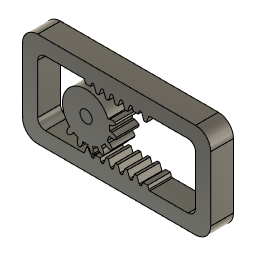
movement-114 v32 (Autodesk Fusion 360 design; units mm, degrees)
description: Spur Gear; Module: 2.0; Num Teeth: 18; Pressure Angle: 20.0; Backlash: 0.15 mm
Autodesk Fusion 360 part; units mm, degrees
note: some values were not read from the file. Set by a fixed rule: which face or edge a step refers to.
sketch "rack-side" plane through (0, 0, 0) normal (0, 1, 0) x (1, 0, 0)
  line L0 (0, 0) -> (43.9823, 0)
  line L1 (43.9823, 0) -> (43.9823, -10)
  line L2 (43.9823, -10) -> (0, -10)
  line L3 (0, -10) -> (0, 0)
  line L4 (0, -12.5) -> (43.9823, -12.5) construction
  line L5 (0, -14.5) -> (43.9823, -14.5) construction
  line L6 (0.6609, -10) -> (2.2987, -14.5)
  line L7 (2.2987, -14.5) -> (3.9844, -14.5)
  line L8 (3.9844, -14.5) -> (5.6223, -10)
  line L9 (0, -31.25) -> (43.9823, -31.25) construction
  point P0 (1.5708, -12.5)
  point P1 (4.7124, -12.5)
  point P2 (3.1416, -14.5)
  point P3 (21.9911, -31.25)
  dimension "d8" = 43.9823
  dimension "d9" = 10
  dimension "d10" = 2.5
  dimension "d11" = 2
  dimension "d12" = 70
  dimension "d13" = 3.1416
  dimension "d14" = 3.1416
  dimension "d32" = 18.75
  constraint horizontal L0
  constraint vertical L1
  constraint horizontal L2
  constraint vertical L3
  constraint coincident L0.start L3.end
  constraint coincident L3 L5.start
  constraint coincident L3 L4.start
  constraint equal L2 L4
  constraint equal L2 L5
  constraint coincident L2 L6.start
  constraint coincident L5 L6.end
  constraint coincident L5 L7.end
  constraint coincident L2 L8.end
  constraint equal L6 L8
  constraint coincident L4 P0
  constraint coincident L6 P0
  constraint coincident L8 P1
  constraint coincident L4 P1
  constraint midpoint L7 P2
  constraint horizontal L9
  constraint coincident L3 L9.start
  constraint equal L0 L9
  constraint midpoint L9 P3
  measures "d8" distance of L0.start L0.end
  measures "d9" distance of L0.start L2.end
  measures "d10" distance of L2 L4
  measures "d11" distance of L4 L5
  measures "d12" angle of L2 L6
  measures "d13" distance of P0 P1
  measures "d14" distance of L3 P2
  measures "d32" distance of L4 L9
extrude "Extrude1" add sketch "rack-side" along normal blind 15 contours L0 L1 L2 L3 makes body 1
extrude "Extrude2" add sketch "rack-side" along normal blind 15 contours L2 L6 L7 L8 bodies 1
fillet "Fillet1" radius 0.76 2 edges at (0.6609, 7.5, 10) (5.6223, 7.5, 10) on bodies 1
pattern_linear "R-Pattern1" count 7 spacing 6.2832 along (1, 0, 0) of "Extrude2", "Fillet1"
copy_body "Body->Comp1" bodies 1 removing the originals makes body 2 in component "rack"
ref_plane "WorkPlane1" through (21.9911, 7.5, 5) normal (-1, 0, 0) x (0, 0, 1) in component "rack"
ref_plane "WorkPlane2" through (21.9911, 0, 31.25) normal (0, 0, 1) x (1, 0, 0) in component "rack"
extrude "Extrude1'" add 1 faces at (0, 5, 6.6667) along direction (-1, 0, 0) blind 40 on bodies 2 bodies 2 in component "rack"
mirror "Mirror1" about plane through (21.9911, 7.5, 5) normal (-1, 0, 0) of "Extrude1'" in component "rack"
mirror "Mirror2" about plane through (21.9911, 0, 31.25) normal (0, 0, 1) of bodies 2 makes body 3 in component "rack"
sketch "rack-top" plane through (0, 0, 10) normal (0, 0, 1) x (-1, 0, 0)
  line L0 (-0.1287, 0) -> (-0.1287, -15)
  line L1 (-0.1287, -15) -> (40, -15)
  line L2 (40, -15) -> (40, 0)
  line L3 (40, 0) -> (-0.1287, 0)
  line L4 (-0.1287, -15) -> (40, -15)
  line L5 (40, 0) -> (40, -15)
  line L6 (-0.1287, -15) -> (-0.1287, 0)
  line L7 (-0.1287, 0) -> (40, 0)
  line L8 (30, -15) -> (30, 0)
  dimension "d35" = 10
  constraint coincident L4 L8.start
  constraint coincident L7 L8.end
  constraint perpendicular L7 L8
  measures "d35" distance of L5 L8
extrude "Extrude2'" add sketch "rack-top" along normal up to surface (42.5 mm away) contours L1 L2 L3 L4 L5 L7 L8 bodies 2 3 in component "rack"
mirror "Mirror3" about plane through (21.9911, 7.5, 5) normal (-1, 0, 0) of "Extrude2'" in component "rack"
fillet "Fillet1'" radius 10 4 edges at (83.9823, 7.5, 62.5) (83.9823, 7.5, 0) (-40, 7.5, 0) (-40, 7.5, 62.5) on bodies 2 in component "rack"
fillet "Fillet2" radius 5 4 edges at (73.9823, 7.5, 10) (73.9823, 7.5, 52.5) (-30, 7.5, 52.5) (-30, 7.5, 10) on bodies 2 in component "rack"
ref_plane "WorkPlane3" through (21.9911, 7.5, 31.25) normal (0, 0, 1) x (-1, 0, 0)
sketch "Sketch1" plane through (0, 0, 0) normal (0, 0, 1) x (1, 0, 0) in component "spur-gear"
  circle A0 centre (0, 0) radius 15.5492
extrude "Extrude1''" add sketch "Sketch1" along normal blind 15 separate body makes body 4 in component "spur-gear"
sketch "Sketch2" plane through (0, 0, 0) normal (0, 0, 1) x (1, 0, 0) in component "spur-gear"
  spline S0 degree 5 poles (16.8298, -1.6901) (16.8389, -1.691) (16.8569, -1.6926) (16.8841, -1.6941) (16.9204, -1.6949) (16.9658, -1.6938) (17.0113, -1.6914) (17.0569, -1.6881) (17.1025, -1.6843) (17.1481, -1.6802) (17.1937, -1.6757) (17.2394, -1.6708) (17.2851, -1.6653) (17.3308, -1.6592) (17.3764, -1.6524) (17.4221, -1.6449) (17.4678, -1.6369) (17.5136, -1.6284) (17.5593, -1.6195) (17.605, -1.6103) (17.6507, -1.6007) (17.6963, -1.5906) (17.742, -1.5802) (17.7877, -1.5693) (17.8334, -1.5581) (17.879, -1.5464) (17.9246, -1.5343) (17.9703, -1.5218) (18.0159, -1.509) (18.0614, -1.4958) (18.107, -1.4823) (18.1525, -1.4685) (18.1981, -1.4543) (18.2436, -1.4397) (18.289, -1.4249) (18.3345, -1.4096) (18.3799, -1.3941) (18.4253, -1.3782) (18.4707, -1.362) (18.516, -1.3455) (18.5613, -1.3287) (18.6066, -1.3116) (18.6518, -1.2941) (18.697, -1.2764) (18.7422, -1.2584) (18.7874, -1.24) (18.8325, -1.2214) (18.8775, -1.2024) (18.9226, -1.1832) (18.9676, -1.1637) (19.0125, -1.1439) (19.0574, -1.1238) (19.1023, -1.1035) (19.1471, -1.0828) (19.1919, -1.0619) (19.2367, -1.0407) (19.2814, -1.0192) (19.326, -0.9975) (19.3706, -0.9755) (19.4152, -0.9532) (19.4597, -0.9307) (19.5041, -0.9079) (19.5485, -0.8848) (19.5929, -0.8615) (19.6372, -0.8379) (19.6815, -0.814) (19.7257, -0.7899) (19.7698, -0.7655) (19.8139, -0.7409) (19.858, -0.7161) (19.902, -0.6909) (19.9371, -0.6706) (19.9634, -0.6553) (19.981, -0.645) (19.9898, -0.6399) knots 0 0 0 0 0 0 0.01428571 0.02857143 0.04285714 0.05714286 0.07142857 0.08571429 0.1 0.11428571 0.12857143 0.14285714 0.15714286 0.17142857 0.18571429 0.2 0.21428571 0.22857143 0.24285714 0.25714286 0.27142857 0.28571429 0.3 0.31428571 0.32857143 0.34285714 0.35714286 0.37142857 0.38571429 0.4 0.41428571 0.42857143 0.44285714 0.45714286 0.47142857 0.48571429 0.5 0.51428571 0.52857143 0.54285714 0.55714286 0.57142857 0.58571429 0.6 0.61428571 0.62857143 0.64285714 0.65714286 0.67142857 0.68571429 0.7 0.71428571 0.72857143 0.74285714 0.75714286 0.77142857 0.78571429 0.8 0.81428571 0.82857143 0.84285714 0.85714286 0.87142857 0.88571429 0.9 0.91428571 0.92857143 0.94285714 0.95714286 0.97142857 0.98571429 1 1 1 1 1 1
  spline S1 degree 5 poles (16.8298, 1.6901) (16.8389, 1.691) (16.8569, 1.6926) (16.8841, 1.6941) (16.9204, 1.6949) (16.9658, 1.6938) (17.0113, 1.6914) (17.0569, 1.6881) (17.1025, 1.6843) (17.1481, 1.6802) (17.1937, 1.6757) (17.2394, 1.6708) (17.2851, 1.6653) (17.3308, 1.6592) (17.3764, 1.6524) (17.4221, 1.6449) (17.4678, 1.6369) (17.5136, 1.6284) (17.5593, 1.6195) (17.605, 1.6103) (17.6507, 1.6007) (17.6963, 1.5906) (17.742, 1.5802) (17.7877, 1.5693) (17.8334, 1.5581) (17.879, 1.5464) (17.9246, 1.5343) (17.9703, 1.5218) (18.0159, 1.509) (18.0614, 1.4958) (18.107, 1.4823) (18.1525, 1.4685) (18.1981, 1.4543) (18.2436, 1.4397) (18.289, 1.4249) (18.3345, 1.4096) (18.3799, 1.3941) (18.4253, 1.3782) (18.4707, 1.362) (18.516, 1.3455) (18.5613, 1.3287) (18.6066, 1.3116) (18.6518, 1.2941) (18.697, 1.2764) (18.7422, 1.2584) (18.7874, 1.24) (18.8325, 1.2214) (18.8775, 1.2024) (18.9226, 1.1832) (18.9676, 1.1637) (19.0125, 1.1439) (19.0574, 1.1238) (19.1023, 1.1035) (19.1471, 1.0828) (19.1919, 1.0619) (19.2367, 1.0407) (19.2814, 1.0192) (19.326, 0.9975) (19.3706, 0.9755) (19.4152, 0.9532) (19.4597, 0.9307) (19.5041, 0.9079) (19.5485, 0.8848) (19.5929, 0.8615) (19.6372, 0.8379) (19.6815, 0.814) (19.7257, 0.7899) (19.7698, 0.7655) (19.8139, 0.7409) (19.858, 0.7161) (19.902, 0.6909) (19.9371, 0.6706) (19.9634, 0.6553) (19.981, 0.645) (19.9898, 0.6399) knots 0 0 0 0 0 0 0.01428571 0.02857143 0.04285714 0.05714286 0.07142857 0.08571429 0.1 0.11428571 0.12857143 0.14285714 0.15714286 0.17142857 0.18571429 0.2 0.21428571 0.22857143 0.24285714 0.25714286 0.27142857 0.28571429 0.3 0.31428571 0.32857143 0.34285714 0.35714286 0.37142857 0.38571429 0.4 0.41428571 0.42857143 0.44285714 0.45714286 0.47142857 0.48571429 0.5 0.51428571 0.52857143 0.54285714 0.55714286 0.57142857 0.58571429 0.6 0.61428571 0.62857143 0.64285714 0.65714286 0.67142857 0.68571429 0.7 0.71428571 0.72857143 0.74285714 0.75714286 0.77142857 0.78571429 0.8 0.81428571 0.82857143 0.84285714 0.85714286 0.87142857 0.88571429 0.9 0.91428571 0.92857143 0.94285714 0.95714286 0.97142857 0.98571429 1 1 1 1 1 1
  arc A0 (19.9898, -0.6399) -> (19.9898, 0.6399) centre (0, 0) ccw
  line L0 (15.4614, -1.5537) -> (16.8298, -1.6901)
  line L1 (15.4614, 1.5537) -> (16.8298, 1.6901)
  line L2 (15.4614, -1.5537) -> (15.4614, 1.5537)
  point P0 (17.0515, -1.6884)
  point P1 (17.2751, -1.6664)
  point P2 (17.4998, -1.6309)
  point P3 (17.7254, -1.5839)
  point P4 (17.9516, -1.5269)
  point P5 (18.1783, -1.4604)
  point P6 (18.4052, -1.3852)
  point P7 (18.6322, -1.3017)
  point P8 (18.8592, -1.2101)
  point P9 (19.0861, -1.1108)
  point P10 (19.3127, -1.0039)
  point P11 (19.539, -0.8897)
  point P12 (19.7647, -0.7683)
  point P13 (17.0515, 1.6884)
  point P14 (17.2751, 1.6664)
  point P15 (17.4998, 1.6309)
  point P16 (17.7254, 1.5839)
  point P17 (17.9516, 1.5269)
  point P18 (18.1783, 1.4604)
  point P19 (18.4052, 1.3852)
  point P20 (18.6322, 1.3017)
  point P21 (18.8592, 1.2101)
  point P22 (19.0861, 1.1108)
  point P23 (19.3127, 1.0039)
  point P24 (19.539, 0.8897)
  point P25 (19.7647, 0.7683)
extrude "Extrude2''" add sketch "Sketch2" along normal blind 15 bodies 4 in component "spur-gear"
pattern_circular "C-Pattern1" count 15 over 360 about axis through (0, 0, 0) along (0, 0, 1) of "Extrude2''" in component "spur-gear"
sketch "Sketch3" plane through (0, 0, 0) normal (0, 0, 1) x (1, 0, 0) in component "spur-gear"
  circle A0 centre (0, 0) radius 18 construction
  circle A1 centre (0, 0) radius 4
  dimension "d73_1" = 8
  constraint concentric A0 A1
  constraint coincident A0.centre A1.centre
  measures "d73_1" diameter of A1
extrude "Extrude3" cut sketch "Sketch3" along normal through all bodies 4 in component "spur-gear"
sketch "Sketch1 (2)" plane through (0, 0, 0) normal (0, 1, 0) x (1, 0, 0) in component "shaft"
  circle A0 centre (4.7674, -31.1301) radius 4
extrude "Extrude1'''" add sketch "Sketch1 (2)" along normal blind 50 separate body makes body 5 in component "shaft"
move_body "Move1" bodies 5 to x (1, 0, 0) y (0, 1, 0) z (0, 0, 1) at (-20, -5, 0) in component "shaft"
move_face "OffsetFaces7" offset -2 4 faces at (40.5598, 5, 14.5) (9.1438, 5, 14.5) (2.8606, 5, 48) (34.2766, 5, 48) on bodies 2 in component "rack"
sketch "Sketch7" plane through (0, 0, 0) normal (0, 0, 1) x (1, 0, 0) in component "spur-gear"
  circle A0 centre (0, 0) radius 15.5492
  line L0 (-14.81, -4.7374) -> (-16.1107, -5.1523)
  spline S0 degree 5 poles (-16.1107, -5.1523) (-16.1193, -5.155) (-16.1367, -5.1603) (-16.1629, -5.1675) (-16.1983, -5.1758) (-16.2429, -5.1842) (-16.2879, -5.1913) (-16.3332, -5.1975) (-16.3786, -5.2033) (-16.4241, -5.2087) (-16.4696, -5.2139) (-16.5153, -5.2186) (-16.5611, -5.2227) (-16.6071, -5.2262) (-16.6532, -5.229) (-16.6994, -5.2312) (-16.7458, -5.2329) (-16.7923, -5.2341) (-16.8388, -5.2349) (-16.8855, -5.2354) (-16.9322, -5.2355) (-16.9789, -5.2352) (-17.0258, -5.2344) (-17.0727, -5.2333) (-17.1197, -5.2318) (-17.1668, -5.2298) (-17.2139, -5.2275) (-17.2612, -5.2248) (-17.3084, -5.2217) (-17.3557, -5.2183) (-17.4031, -5.2146) (-17.4506, -5.2105) (-17.498, -5.2061) (-17.5456, -5.2013) (-17.5931, -5.1962) (-17.6408, -5.1908) (-17.6884, -5.185) (-17.7361, -5.1789) (-17.7839, -5.1725) (-17.8316, -5.1658) (-17.8795, -5.1588) (-17.9273, -5.1514) (-17.9752, -5.1438) (-18.0231, -5.1358) (-18.071, -5.1276) (-18.119, -5.119) (-18.167, -5.1102) (-18.215, -5.101) (-18.2631, -5.0916) (-18.3111, -5.0819) (-18.3592, -5.0718) (-18.4073, -5.0615) (-18.4554, -5.0509) (-18.5036, -5.0401) (-18.5517, -5.0289) (-18.5999, -5.0175) (-18.6481, -5.0058) (-18.6963, -4.9938) (-18.7445, -4.9816) (-18.7927, -4.969) (-18.8409, -4.9562) (-18.8892, -4.9432) (-18.9374, -4.9298) (-18.9857, -4.9162) (-19.0339, -4.9024) (-19.0821, -4.8882) (-19.1304, -4.8738) (-19.1787, -4.8592) (-19.2269, -4.8443) (-19.2752, -4.8291) (-19.3234, -4.8137) (-19.362, -4.8011) (-19.3909, -4.7916) (-19.4102, -4.7852) (-19.4199, -4.782) knots 0 0 0 0 0 0 0.01428571 0.02857143 0.04285714 0.05714286 0.07142857 0.08571429 0.1 0.11428571 0.12857143 0.14285714 0.15714286 0.17142857 0.18571429 0.2 0.21428571 0.22857143 0.24285714 0.25714286 0.27142857 0.28571429 0.3 0.31428571 0.32857143 0.34285714 0.35714286 0.37142857 0.38571429 0.4 0.41428571 0.42857143 0.44285714 0.45714286 0.47142857 0.48571429 0.5 0.51428571 0.52857143 0.54285714 0.55714286 0.57142857 0.58571429 0.6 0.61428571 0.62857143 0.64285714 0.65714286 0.67142857 0.68571429 0.7 0.71428571 0.72857143 0.74285714 0.75714286 0.77142857 0.78571429 0.8 0.81428571 0.82857143 0.84285714 0.85714286 0.87142857 0.88571429 0.9 0.91428571 0.92857143 0.94285714 0.95714286 0.97142857 0.98571429 1 1 1 1 1 1
  arc A1 (-19.686, -3.5302) -> (-19.4199, -4.782) centre (0, 0) ccw
  spline S1 degree 5 poles (-16.8134, -1.8459) (-16.8225, -1.8469) (-16.8405, -1.8492) (-16.8674, -1.8533) (-16.903, -1.8601) (-16.9473, -1.8706) (-16.9913, -1.8824) (-17.0351, -1.8952) (-17.0789, -1.9083) (-17.1227, -1.9219) (-17.1664, -1.9357) (-17.2101, -1.95) (-17.2536, -1.9648) (-17.297, -1.9803) (-17.3403, -1.9965) (-17.3834, -2.0133) (-17.4265, -2.0307) (-17.4694, -2.0485) (-17.5123, -2.0666) (-17.555, -2.0852) (-17.5977, -2.1041) (-17.6403, -2.1234) (-17.6829, -2.1431) (-17.7253, -2.1632) (-17.7676, -2.1838) (-17.8098, -2.2047) (-17.8519, -2.226) (-17.894, -2.2477) (-17.9359, -2.2697) (-17.9778, -2.292) (-18.0195, -2.3147) (-18.0612, -2.3377) (-18.1028, -2.3611) (-18.1442, -2.3848) (-18.1856, -2.4088) (-18.2269, -2.4331) (-18.2681, -2.4578) (-18.3092, -2.4827) (-18.3502, -2.508) (-18.3911, -2.5336) (-18.432, -2.5595) (-18.4727, -2.5856) (-18.5133, -2.6121) (-18.5539, -2.6388) (-18.5943, -2.6659) (-18.6346, -2.6932) (-18.6749, -2.7208) (-18.715, -2.7487) (-18.7551, -2.7769) (-18.795, -2.8053) (-18.8349, -2.834) (-18.8746, -2.863) (-18.9143, -2.8922) (-18.9539, -2.9217) (-18.9933, -2.9515) (-19.0327, -2.9816) (-19.0719, -3.0118) (-19.1111, -3.0424) (-19.1501, -3.0732) (-19.1891, -3.1042) (-19.2279, -3.1356) (-19.2667, -3.1671) (-19.3053, -3.1989) (-19.3439, -3.231) (-19.3823, -3.2633) (-19.4206, -3.2958) (-19.4589, -3.3286) (-19.497, -3.3616) (-19.535, -3.3948) (-19.5729, -3.4283) (-19.6107, -3.462) (-19.6409, -3.4892) (-19.6634, -3.5096) (-19.6785, -3.5233) (-19.686, -3.5302) knots 0 0 0 0 0 0 0.01428571 0.02857143 0.04285714 0.05714286 0.07142857 0.08571429 0.1 0.11428571 0.12857143 0.14285714 0.15714286 0.17142857 0.18571429 0.2 0.21428571 0.22857143 0.24285714 0.25714286 0.27142857 0.28571429 0.3 0.31428571 0.32857143 0.34285714 0.35714286 0.37142857 0.38571429 0.4 0.41428571 0.42857143 0.44285714 0.45714286 0.47142857 0.48571429 0.5 0.51428571 0.52857143 0.54285714 0.55714286 0.57142857 0.58571429 0.6 0.61428571 0.62857143 0.64285714 0.65714286 0.67142857 0.68571429 0.7 0.71428571 0.72857143 0.74285714 0.75714286 0.77142857 0.78571429 0.8 0.81428571 0.82857143 0.84285714 0.85714286 0.87142857 0.88571429 0.9 0.91428571 0.92857143 0.94285714 0.95714286 0.97142857 0.98571429 1 1 1 1 1 1
  line L1 (-15.4564, -1.696) -> (-16.8134, -1.8459)
  line L2 (-15.4564, 1.696) -> (-16.8134, 1.8459)
  spline S2 degree 5 poles (-16.8134, 1.8459) (-16.8225, 1.8469) (-16.8405, 1.8492) (-16.8674, 1.8533) (-16.903, 1.8601) (-16.9473, 1.8706) (-16.9913, 1.8824) (-17.0351, 1.8952) (-17.0789, 1.9083) (-17.1227, 1.9219) (-17.1664, 1.9357) (-17.2101, 1.95) (-17.2536, 1.9648) (-17.297, 1.9803) (-17.3403, 1.9965) (-17.3834, 2.0133) (-17.4265, 2.0307) (-17.4694, 2.0485) (-17.5123, 2.0666) (-17.555, 2.0852) (-17.5977, 2.1041) (-17.6403, 2.1234) (-17.6829, 2.1431) (-17.7253, 2.1632) (-17.7676, 2.1838) (-17.8098, 2.2047) (-17.8519, 2.226) (-17.894, 2.2477) (-17.9359, 2.2697) (-17.9778, 2.292) (-18.0195, 2.3147) (-18.0612, 2.3377) (-18.1028, 2.3611) (-18.1442, 2.3848) (-18.1856, 2.4088) (-18.2269, 2.4331) (-18.2681, 2.4578) (-18.3092, 2.4827) (-18.3502, 2.508) (-18.3911, 2.5336) (-18.432, 2.5595) (-18.4727, 2.5856) (-18.5133, 2.6121) (-18.5539, 2.6388) (-18.5943, 2.6659) (-18.6346, 2.6932) (-18.6749, 2.7208) (-18.715, 2.7487) (-18.7551, 2.7769) (-18.795, 2.8053) (-18.8349, 2.834) (-18.8746, 2.863) (-18.9143, 2.8922) (-18.9539, 2.9217) (-18.9933, 2.9515) (-19.0327, 2.9816) (-19.0719, 3.0118) (-19.1111, 3.0424) (-19.1501, 3.0732) (-19.1891, 3.1042) (-19.2279, 3.1356) (-19.2667, 3.1671) (-19.3053, 3.1989) (-19.3439, 3.231) (-19.3823, 3.2633) (-19.4206, 3.2958) (-19.4589, 3.3286) (-19.497, 3.3616) (-19.535, 3.3948) (-19.5729, 3.4283) (-19.6107, 3.462) (-19.6409, 3.4892) (-19.6634, 3.5096) (-19.6785, 3.5233) (-19.686, 3.5302) knots 0 0 0 0 0 0 0.01428571 0.02857143 0.04285714 0.05714286 0.07142857 0.08571429 0.1 0.11428571 0.12857143 0.14285714 0.15714286 0.17142857 0.18571429 0.2 0.21428571 0.22857143 0.24285714 0.25714286 0.27142857 0.28571429 0.3 0.31428571 0.32857143 0.34285714 0.35714286 0.37142857 0.38571429 0.4 0.41428571 0.42857143 0.44285714 0.45714286 0.47142857 0.48571429 0.5 0.51428571 0.52857143 0.54285714 0.55714286 0.57142857 0.58571429 0.6 0.61428571 0.62857143 0.64285714 0.65714286 0.67142857 0.68571429 0.7 0.71428571 0.72857143 0.74285714 0.75714286 0.77142857 0.78571429 0.8 0.81428571 0.82857143 0.84285714 0.85714286 0.87142857 0.88571429 0.9 0.91428571 0.92857143 0.94285714 0.95714286 0.97142857 0.98571429 1 1 1 1 1 1
  arc A2 (-19.4199, 4.782) -> (-19.686, 3.5302) centre (0, 0) ccw
  spline S3 degree 5 poles (-16.1107, 5.1523) (-16.1193, 5.155) (-16.1367, 5.1603) (-16.1629, 5.1675) (-16.1983, 5.1758) (-16.2429, 5.1842) (-16.2879, 5.1913) (-16.3332, 5.1975) (-16.3786, 5.2033) (-16.4241, 5.2087) (-16.4696, 5.2139) (-16.5153, 5.2186) (-16.5611, 5.2227) (-16.6071, 5.2262) (-16.6532, 5.229) (-16.6994, 5.2312) (-16.7458, 5.2329) (-16.7923, 5.2341) (-16.8388, 5.2349) (-16.8855, 5.2354) (-16.9322, 5.2355) (-16.9789, 5.2352) (-17.0258, 5.2344) (-17.0727, 5.2333) (-17.1197, 5.2318) (-17.1668, 5.2298) (-17.2139, 5.2275) (-17.2612, 5.2248) (-17.3084, 5.2217) (-17.3557, 5.2183) (-17.4031, 5.2146) (-17.4506, 5.2105) (-17.498, 5.2061) (-17.5456, 5.2013) (-17.5931, 5.1962) (-17.6408, 5.1908) (-17.6884, 5.185) (-17.7361, 5.1789) (-17.7839, 5.1725) (-17.8316, 5.1658) (-17.8795, 5.1588) (-17.9273, 5.1514) (-17.9752, 5.1438) (-18.0231, 5.1358) (-18.071, 5.1276) (-18.119, 5.119) (-18.167, 5.1102) (-18.215, 5.101) (-18.2631, 5.0916) (-18.3111, 5.0819) (-18.3592, 5.0718) (-18.4073, 5.0615) (-18.4554, 5.0509) (-18.5036, 5.0401) (-18.5517, 5.0289) (-18.5999, 5.0175) (-18.6481, 5.0058) (-18.6963, 4.9938) (-18.7445, 4.9816) (-18.7927, 4.969) (-18.8409, 4.9562) (-18.8892, 4.9432) (-18.9374, 4.9298) (-18.9857, 4.9162) (-19.0339, 4.9024) (-19.0821, 4.8882) (-19.1304, 4.8738) (-19.1787, 4.8592) (-19.2269, 4.8443) (-19.2752, 4.8291) (-19.3234, 4.8137) (-19.362, 4.8011) (-19.3909, 4.7916) (-19.4102, 4.7852) (-19.4199, 4.782) knots 0 0 0 0 0 0 0.01428571 0.02857143 0.04285714 0.05714286 0.07142857 0.08571429 0.1 0.11428571 0.12857143 0.14285714 0.15714286 0.17142857 0.18571429 0.2 0.21428571 0.22857143 0.24285714 0.25714286 0.27142857 0.28571429 0.3 0.31428571 0.32857143 0.34285714 0.35714286 0.37142857 0.38571429 0.4 0.41428571 0.42857143 0.44285714 0.45714286 0.47142857 0.48571429 0.5 0.51428571 0.52857143 0.54285714 0.55714286 0.57142857 0.58571429 0.6 0.61428571 0.62857143 0.64285714 0.65714286 0.67142857 0.68571429 0.7 0.71428571 0.72857143 0.74285714 0.75714286 0.77142857 0.78571429 0.8 0.81428571 0.82857143 0.84285714 0.85714286 0.87142857 0.88571429 0.9 0.91428571 0.92857143 0.94285714 0.95714286 0.97142857 0.98571429 1 1 1 1 1 1
  line L3 (-14.81, 4.7374) -> (-16.1107, 5.1523)
  line L4 (-13.4303, 7.836) -> (-14.609, 8.525)
  spline S4 degree 5 poles (-14.609, 8.525) (-14.6169, 8.5296) (-14.6324, 8.539) (-14.6553, 8.5536) (-14.6851, 8.5744) (-14.7212, 8.6019) (-14.7566, 8.6307) (-14.7915, 8.6601) (-14.8262, 8.69) (-14.8607, 8.7201) (-14.895, 8.7506) (-14.929, 8.7813) (-14.9628, 8.8126) (-14.9961, 8.8444) (-15.0291, 8.8768) (-15.0616, 8.9097) (-15.0939, 8.9431) (-15.1259, 8.9768) (-15.1577, 9.0108) (-15.1892, 9.0452) (-15.2205, 9.0798) (-15.2516, 9.1148) (-15.2824, 9.1501) (-15.313, 9.1857) (-15.3433, 9.2217) (-15.3733, 9.258) (-15.4032, 9.2946) (-15.4327, 9.3315) (-15.4621, 9.3686) (-15.4912, 9.4061) (-15.5202, 9.4438) (-15.5489, 9.4818) (-15.5774, 9.52) (-15.6056, 9.5585) (-15.6337, 9.5973) (-15.6615, 9.6363) (-15.6891, 9.6756) (-15.7165, 9.7151) (-15.7437, 9.7549) (-15.7706, 9.7949) (-15.7974, 9.8351) (-15.824, 9.8756) (-15.8503, 9.9163) (-15.8765, 9.9572) (-15.9024, 9.9984) (-15.9282, 10.0397) (-15.9537, 10.0813) (-15.979, 10.1231) (-16.0042, 10.1652) (-16.0291, 10.2074) (-16.0538, 10.2498) (-16.0784, 10.2925) (-16.1027, 10.3353) (-16.1268, 10.3784) (-16.1508, 10.4216) (-16.1745, 10.4651) (-16.198, 10.5087) (-16.2214, 10.5525) (-16.2445, 10.5966) (-16.2675, 10.6408) (-16.2902, 10.6852) (-16.3128, 10.7298) (-16.3352, 10.7745) (-16.3574, 10.8195) (-16.3793, 10.8646) (-16.4011, 10.9099) (-16.4227, 10.9554) (-16.4441, 11.0011) (-16.4653, 11.0469) (-16.4863, 11.0929) (-16.5072, 11.1391) (-16.5237, 11.1762) (-16.5359, 11.2041) (-16.5441, 11.2227) (-16.5482, 11.232) knots 0 0 0 0 0 0 0.01428571 0.02857143 0.04285714 0.05714286 0.07142857 0.08571429 0.1 0.11428571 0.12857143 0.14285714 0.15714286 0.17142857 0.18571429 0.2 0.21428571 0.22857143 0.24285714 0.25714286 0.27142857 0.28571429 0.3 0.31428571 0.32857143 0.34285714 0.35714286 0.37142857 0.38571429 0.4 0.41428571 0.42857143 0.44285714 0.45714286 0.47142857 0.48571429 0.5 0.51428571 0.52857143 0.54285714 0.55714286 0.57142857 0.58571429 0.6 0.61428571 0.62857143 0.64285714 0.65714286 0.67142857 0.68571429 0.7 0.71428571 0.72857143 0.74285714 0.75714286 0.77142857 0.78571429 0.8 0.81428571 0.82857143 0.84285714 0.85714286 0.87142857 0.88571429 0.9 0.91428571 0.92857143 0.94285714 0.95714286 0.97142857 0.98571429 1 1 1 1 1 1
  arc A3 (-15.7959, 12.2674) -> (-16.5482, 11.232) centre (0, 0) ccw
  spline S5 degree 5 poles (-12.6222, 11.2596) (-12.629, 11.2657) (-12.6427, 11.2776) (-12.6637, 11.2948) (-12.6927, 11.3167) (-12.73, 11.3426) (-12.7683, 11.3674) (-12.8071, 11.3915) (-12.8462, 11.4152) (-12.8855, 11.4387) (-12.9251, 11.4619) (-12.9649, 11.4848) (-13.0051, 11.5072) (-13.0456, 11.5291) (-13.0866, 11.5504) (-13.128, 11.5712) (-13.1697, 11.5916) (-13.2116, 11.6116) (-13.2538, 11.6313) (-13.2962, 11.6507) (-13.3388, 11.6698) (-13.3817, 11.6885) (-13.4248, 11.7069) (-13.4681, 11.725) (-13.5117, 11.7427) (-13.5555, 11.76) (-13.5995, 11.7771) (-13.6437, 11.7938) (-13.6882, 11.8103) (-13.7328, 11.8264) (-13.7776, 11.8423) (-13.8226, 11.8578) (-13.8677, 11.8731) (-13.9131, 11.8881) (-13.9586, 11.9028) (-14.0043, 11.9172) (-14.0502, 11.9313) (-14.0963, 11.9451) (-14.1425, 11.9587) (-14.1889, 11.972) (-14.2354, 11.985) (-14.2821, 11.9978) (-14.329, 12.0103) (-14.376, 12.0225) (-14.4231, 12.0344) (-14.4704, 12.0461) (-14.5179, 12.0576) (-14.5655, 12.0687) (-14.6132, 12.0797) (-14.6611, 12.0903) (-14.7091, 12.1007) (-14.7572, 12.1109) (-14.8055, 12.1208) (-14.8539, 12.1304) (-14.9024, 12.1398) (-14.9511, 12.149) (-14.9998, 12.1579) (-15.0487, 12.1665) (-15.0978, 12.175) (-15.1469, 12.1831) (-15.1962, 12.191) (-15.2455, 12.1987) (-15.295, 12.2062) (-15.3446, 12.2134) (-15.3944, 12.2203) (-15.4442, 12.227) (-15.4941, 12.2335) (-15.5442, 12.2398) (-15.5943, 12.2458) (-15.6446, 12.2515) (-15.6949, 12.2571) (-15.7353, 12.2613) (-15.7656, 12.2644) (-15.7858, 12.2664) (-15.7959, 12.2674) knots 0 0 0 0 0 0 0.01428571 0.02857143 0.04285714 0.05714286 0.07142857 0.08571429 0.1 0.11428571 0.12857143 0.14285714 0.15714286 0.17142857 0.18571429 0.2 0.21428571 0.22857143 0.24285714 0.25714286 0.27142857 0.28571429 0.3 0.31428571 0.32857143 0.34285714 0.35714286 0.37142857 0.38571429 0.4 0.41428571 0.42857143 0.44285714 0.45714286 0.47142857 0.48571429 0.5 0.51428571 0.52857143 0.54285714 0.55714286 0.57142857 0.58571429 0.6 0.61428571 0.62857143 0.64285714 0.65714286 0.67142857 0.68571429 0.7 0.71428571 0.72857143 0.74285714 0.75714286 0.77142857 0.78571429 0.8 0.81428571 0.82857143 0.84285714 0.85714286 0.87142857 0.88571429 0.9 0.91428571 0.92857143 0.94285714 0.95714286 0.97142857 0.98571429 1 1 1 1 1 1
  line L5 (-11.6027, 10.3515) -> (-12.6222, 11.2596)
  line L6 (-9.082, 12.6212) -> (-9.8786, 13.73)
  spline S6 degree 5 poles (-9.8786, 13.73) (-9.8839, 13.7374) (-9.8943, 13.7523) (-9.9092, 13.775) (-9.928, 13.8061) (-9.9498, 13.8459) (-9.9704, 13.8866) (-9.9904, 13.9277) (-10.0099, 13.9691) (-10.0291, 14.0106) (-10.0481, 14.0524) (-10.0667, 14.0944) (-10.0848, 14.1366) (-10.1023, 14.1793) (-10.1192, 14.2223) (-10.1356, 14.2656) (-10.1515, 14.3092) (-10.167, 14.353) (-10.1822, 14.397) (-10.197, 14.4412) (-10.2115, 14.4856) (-10.2257, 14.5302) (-10.2395, 14.5749) (-10.2529, 14.6199) (-10.266, 14.6651) (-10.2787, 14.7105) (-10.291, 14.7561) (-10.3031, 14.8018) (-10.3148, 14.8477) (-10.3262, 14.8937) (-10.3372, 14.94) (-10.348, 14.9863) (-10.3585, 15.0328) (-10.3686, 15.0795) (-10.3785, 15.1263) (-10.388, 15.1733) (-10.3973, 15.2204) (-10.4062, 15.2677) (-10.4149, 15.3151) (-10.4233, 15.3626) (-10.4313, 15.4102) (-10.4392, 15.458) (-10.4467, 15.5059) (-10.4539, 15.5539) (-10.4609, 15.6021) (-10.4676, 15.6503) (-10.474, 15.6987) (-10.4801, 15.7472) (-10.486, 15.7958) (-10.4916, 15.8445) (-10.4969, 15.8934) (-10.502, 15.9423) (-10.5068, 15.9913) (-10.5113, 16.0405) (-10.5156, 16.0897) (-10.5196, 16.1391) (-10.5234, 16.1885) (-10.5269, 16.2381) (-10.5301, 16.2877) (-10.5331, 16.3374) (-10.5358, 16.3872) (-10.5383, 16.4371) (-10.5405, 16.4871) (-10.5425, 16.5372) (-10.5442, 16.5874) (-10.5457, 16.6377) (-10.5469, 16.688) (-10.5479, 16.7384) (-10.5486, 16.7889) (-10.5491, 16.8395) (-10.5494, 16.8901) (-10.5494, 16.9307) (-10.5492, 16.9612) (-10.5491, 16.9815) (-10.549, 16.9917) knots 0 0 0 0 0 0 0.01428571 0.02857143 0.04285714 0.05714286 0.07142857 0.08571429 0.1 0.11428571 0.12857143 0.14285714 0.15714286 0.17142857 0.18571429 0.2 0.21428571 0.22857143 0.24285714 0.25714286 0.27142857 0.28571429 0.3 0.31428571 0.32857143 0.34285714 0.35714286 0.37142857 0.38571429 0.4 0.41428571 0.42857143 0.44285714 0.45714286 0.47142857 0.48571429 0.5 0.51428571 0.52857143 0.54285714 0.55714286 0.57142857 0.58571429 0.6 0.61428571 0.62857143 0.64285714 0.65714286 0.67142857 0.68571429 0.7 0.71428571 0.72857143 0.74285714 0.75714286 0.77142857 0.78571429 0.8 0.81428571 0.82857143 0.84285714 0.85714286 0.87142857 0.88571429 0.9 0.91428571 0.92857143 0.94285714 0.95714286 0.97142857 0.98571429 1 1 1 1 1 1
  arc A4 (-9.4407, 17.6316) -> (-10.549, 16.9917) centre (0, 0) ccw
  spline S7 degree 5 poles (-6.9512, 15.4201) (-6.955, 15.4284) (-6.9627, 15.4448) (-6.9749, 15.4691) (-6.9924, 15.5009) (-7.016, 15.5397) (-7.0409, 15.5779) (-7.0665, 15.6157) (-7.0926, 15.6533) (-7.119, 15.6908) (-7.1457, 15.7281) (-7.1727, 15.7652) (-7.2003, 15.802) (-7.2285, 15.8385) (-7.2572, 15.8746) (-7.2866, 15.9105) (-7.3164, 15.946) (-7.3465, 15.9814) (-7.3771, 16.0165) (-7.4079, 16.0515) (-7.4391, 16.0862) (-7.4706, 16.1208) (-7.5025, 16.1551) (-7.5348, 16.1893) (-7.5674, 16.2232) (-7.6003, 16.2568) (-7.6336, 16.2903) (-7.6672, 16.3236) (-7.7011, 16.3567) (-7.7353, 16.3896) (-7.7698, 16.4223) (-7.8045, 16.4548) (-7.8396, 16.4871) (-7.8749, 16.5193) (-7.9106, 16.5512) (-7.9465, 16.583) (-7.9826, 16.6145) (-8.0191, 16.6459) (-8.0558, 16.6771) (-8.0928, 16.7081) (-8.13, 16.7389) (-8.1674, 16.7696) (-8.2052, 16.8) (-8.2431, 16.8303) (-8.2813, 16.8604) (-8.3198, 16.8903) (-8.3585, 16.9201) (-8.3974, 16.9497) (-8.4366, 16.979) (-8.476, 17.0082) (-8.5156, 17.0373) (-8.5554, 17.0661) (-8.5955, 17.0948) (-8.6358, 17.1233) (-8.6763, 17.1516) (-8.717, 17.1798) (-8.758, 17.2078) (-8.7991, 17.2356) (-8.8405, 17.2632) (-8.8821, 17.2906) (-8.9238, 17.3179) (-8.9658, 17.345) (-9.008, 17.3719) (-9.0504, 17.3987) (-9.093, 17.4253) (-9.1358, 17.4517) (-9.1788, 17.4779) (-9.2219, 17.504) (-9.2653, 17.5298) (-9.3089, 17.5555) (-9.3526, 17.5811) (-9.3878, 17.6014) (-9.4142, 17.6165) (-9.4319, 17.6266) (-9.4407, 17.6316) knots 0 0 0 0 0 0 0.01428571 0.02857143 0.04285714 0.05714286 0.07142857 0.08571429 0.1 0.11428571 0.12857143 0.14285714 0.15714286 0.17142857 0.18571429 0.2 0.21428571 0.22857143 0.24285714 0.25714286 0.27142857 0.28571429 0.3 0.31428571 0.32857143 0.34285714 0.35714286 0.37142857 0.38571429 0.4 0.41428571 0.42857143 0.44285714 0.45714286 0.47142857 0.48571429 0.5 0.51428571 0.52857143 0.54285714 0.55714286 0.57142857 0.58571429 0.6 0.61428571 0.62857143 0.64285714 0.65714286 0.67142857 0.68571429 0.7 0.71428571 0.72857143 0.74285714 0.75714286 0.77142857 0.78571429 0.8 0.81428571 0.82857143 0.84285714 0.85714286 0.87142857 0.88571429 0.9 0.91428571 0.92857143 0.94285714 0.95714286 0.97142857 0.98571429 1 1 1 1 1 1
  line L7 (-6.3893, 14.1759) -> (-6.9512, 15.4201)
  line L8 (-3.1633, 15.224) -> (-3.44, 16.561)
  spline S8 degree 5 poles (-3.44, 16.561) (-3.4419, 16.5699) (-3.4453, 16.5877) (-3.4497, 16.6145) (-3.4542, 16.6505) (-3.4579, 16.6958) (-3.4603, 16.7414) (-3.4617, 16.787) (-3.4627, 16.8328) (-3.4634, 16.8785) (-3.4638, 16.9244) (-3.4637, 16.9703) (-3.463, 17.0163) (-3.4617, 17.0624) (-3.4596, 17.1085) (-3.457, 17.1548) (-3.4538, 17.2011) (-3.4501, 17.2474) (-3.4461, 17.2938) (-3.4417, 17.3402) (-3.4369, 17.3866) (-3.4317, 17.4331) (-3.4261, 17.4797) (-3.4201, 17.5262) (-3.4136, 17.5728) (-3.4068, 17.6194) (-3.3995, 17.6661) (-3.3919, 17.7127) (-3.3839, 17.7594) (-3.3756, 17.8061) (-3.3669, 17.8529) (-3.3579, 17.8996) (-3.3485, 17.9464) (-3.3388, 17.9931) (-3.3288, 18.0399) (-3.3184, 18.0867) (-3.3077, 18.1335) (-3.2966, 18.1803) (-3.2853, 18.2271) (-3.2736, 18.2739) (-3.2616, 18.3207) (-3.2493, 18.3676) (-3.2367, 18.4144) (-3.2238, 18.4612) (-3.2106, 18.508) (-3.197, 18.5548) (-3.1832, 18.6016) (-3.1691, 18.6484) (-3.1547, 18.6952) (-3.14, 18.742) (-3.125, 18.7888) (-3.1097, 18.8356) (-3.0942, 18.8823) (-3.0783, 18.9291) (-3.0622, 18.9758) (-3.0458, 19.0225) (-3.0291, 19.0692) (-3.0122, 19.1159) (-2.9949, 19.1625) (-2.9774, 19.2092) (-2.9597, 19.2558) (-2.9416, 19.3024) (-2.9233, 19.349) (-2.9048, 19.3955) (-2.8859, 19.4421) (-2.8668, 19.4886) (-2.8475, 19.5351) (-2.8279, 19.5815) (-2.808, 19.6279) (-2.7879, 19.6743) (-2.7675, 19.7207) (-2.751, 19.7578) (-2.7385, 19.7856) (-2.7301, 19.8041) (-2.7259, 19.8134) knots 0 0 0 0 0 0 0.01428571 0.02857143 0.04285714 0.05714286 0.07142857 0.08571429 0.1 0.11428571 0.12857143 0.14285714 0.15714286 0.17142857 0.18571429 0.2 0.21428571 0.22857143 0.24285714 0.25714286 0.27142857 0.28571429 0.3 0.31428571 0.32857143 0.34285714 0.35714286 0.37142857 0.38571429 0.4 0.41428571 0.42857143 0.44285714 0.45714286 0.47142857 0.48571429 0.5 0.51428571 0.52857143 0.54285714 0.55714286 0.57142857 0.58571429 0.6 0.61428571 0.62857143 0.64285714 0.65714286 0.67142857 0.68571429 0.7 0.71428571 0.72857143 0.74285714 0.75714286 0.77142857 0.78571429 0.8 0.81428571 0.82857143 0.84285714 0.85714286 0.87142857 0.88571429 0.9 0.91428571 0.92857143 0.94285714 0.95714286 0.97142857 0.98571429 1 1 1 1 1 1
  arc A5 (-1.4531, 19.9471) -> (-2.7259, 19.8134) centre (0, 0) ccw
  spline S9 degree 5 poles (-0.0784, 16.9143) (-0.0784, 16.9234) (-0.0787, 16.9415) (-0.08, 16.9687) (-0.0831, 17.0049) (-0.0889, 17.0499) (-0.0961, 17.0949) (-0.1041, 17.1399) (-0.1127, 17.1849) (-0.1215, 17.2298) (-0.1307, 17.2747) (-0.1403, 17.3196) (-0.1506, 17.3645) (-0.1615, 17.4092) (-0.173, 17.454) (-0.1852, 17.4986) (-0.198, 17.5433) (-0.2112, 17.5878) (-0.2248, 17.6324) (-0.2388, 17.6768) (-0.2531, 17.7213) (-0.2678, 17.7657) (-0.283, 17.81) (-0.2986, 17.8543) (-0.3146, 17.8985) (-0.331, 17.9427) (-0.3478, 17.9868) (-0.3649, 18.0309) (-0.3824, 18.0749) (-0.4003, 18.1189) (-0.4185, 18.1628) (-0.437, 18.2066) (-0.4559, 18.2504) (-0.4751, 18.2941) (-0.4947, 18.3378) (-0.5146, 18.3814) (-0.5348, 18.4249) (-0.5553, 18.4684) (-0.5761, 18.5119) (-0.5973, 18.5552) (-0.6188, 18.5985) (-0.6405, 18.6418) (-0.6626, 18.6849) (-0.685, 18.728) (-0.7076, 18.7711) (-0.7306, 18.8141) (-0.7538, 18.857) (-0.7774, 18.8998) (-0.8012, 18.9426) (-0.8253, 18.9853) (-0.8497, 19.0279) (-0.8744, 19.0705) (-0.8993, 19.113) (-0.9245, 19.1554) (-0.95, 19.1978) (-0.9758, 19.2401) (-1.0018, 19.2823) (-1.0281, 19.3244) (-1.0546, 19.3665) (-1.0814, 19.4084) (-1.1085, 19.4504) (-1.1358, 19.4922) (-1.1634, 19.5339) (-1.1913, 19.5756) (-1.2194, 19.6172) (-1.2477, 19.6588) (-1.2763, 19.7002) (-1.3052, 19.7416) (-1.3342, 19.7828) (-1.3636, 19.824) (-1.3932, 19.8652) (-1.417, 19.898) (-1.435, 19.9226) (-1.4471, 19.939) (-1.4531, 19.9471) knots 0 0 0 0 0 0 0.01428571 0.02857143 0.04285714 0.05714286 0.07142857 0.08571429 0.1 0.11428571 0.12857143 0.14285714 0.15714286 0.17142857 0.18571429 0.2 0.21428571 0.22857143 0.24285714 0.25714286 0.27142857 0.28571429 0.3 0.31428571 0.32857143 0.34285714 0.35714286 0.37142857 0.38571429 0.4 0.41428571 0.42857143 0.44285714 0.45714286 0.47142857 0.48571429 0.5 0.51428571 0.52857143 0.54285714 0.55714286 0.57142857 0.58571429 0.6 0.61428571 0.62857143 0.64285714 0.65714286 0.67142857 0.68571429 0.7 0.71428571 0.72857143 0.74285714 0.75714286 0.77142857 0.78571429 0.8 0.81428571 0.82857143 0.84285714 0.85714286 0.87142857 0.88571429 0.9 0.91428571 0.92857143 0.94285714 0.95714286 0.97142857 0.98571429 1 1 1 1 1 1
  line L9 (-0.071, 15.549) -> (-0.0784, 16.9143)
  line L10 (3.3023, 15.1945) -> (3.5933, 16.5284)
  spline S10 degree 5 poles (3.5933, 16.5284) (3.5953, 16.5373) (3.5994, 16.5549) (3.6062, 16.5813) (3.6168, 16.616) (3.6318, 16.6589) (3.6482, 16.7014) (3.6654, 16.7437) (3.6831, 16.7859) (3.7011, 16.828) (3.7195, 16.87) (3.7382, 16.912) (3.7575, 16.9537) (3.7775, 16.9952) (3.7981, 17.0366) (3.8194, 17.0777) (3.8411, 17.1187) (3.8633, 17.1596) (3.8858, 17.2003) (3.9088, 17.2409) (3.932, 17.2814) (3.9557, 17.3218) (3.9797, 17.362) (4.0042, 17.4021) (4.029, 17.442) (4.0542, 17.4818) (4.0798, 17.5215) (4.1058, 17.561) (4.1321, 17.6004) (4.1587, 17.6397) (4.1856, 17.6788) (4.2128, 17.7179) (4.2404, 17.7568) (4.2683, 17.7956) (4.2965, 17.8342) (4.325, 17.8727) (4.3538, 17.9111) (4.383, 17.9494) (4.4124, 17.9875) (4.4421, 18.0256) (4.4721, 18.0635) (4.5024, 18.1012) (4.5329, 18.1389) (4.5638, 18.1764) (4.5949, 18.2138) (4.6263, 18.251) (4.658, 18.2882) (4.6899, 18.3252) (4.7221, 18.3621) (4.7545, 18.3988) (4.7873, 18.4355) (4.8202, 18.472) (4.8535, 18.5084) (4.887, 18.5446) (4.9207, 18.5807) (4.9547, 18.6167) (4.9889, 18.6526) (5.0234, 18.6884) (5.0581, 18.724) (5.093, 18.7595) (5.1282, 18.7948) (5.1637, 18.8301) (5.1993, 18.8652) (5.2352, 18.9002) (5.2714, 18.935) (5.3077, 18.9697) (5.3443, 19.0043) (5.3811, 19.0388) (5.4182, 19.0731) (5.4554, 19.1073) (5.4929, 19.1414) (5.5231, 19.1686) (5.5458, 19.1889) (5.561, 19.2024) (5.5686, 19.2091) knots 0 0 0 0 0 0 0.01428571 0.02857143 0.04285714 0.05714286 0.07142857 0.08571429 0.1 0.11428571 0.12857143 0.14285714 0.15714286 0.17142857 0.18571429 0.2 0.21428571 0.22857143 0.24285714 0.25714286 0.27142857 0.28571429 0.3 0.31428571 0.32857143 0.34285714 0.35714286 0.37142857 0.38571429 0.4 0.41428571 0.42857143 0.44285714 0.45714286 0.47142857 0.48571429 0.5 0.51428571 0.52857143 0.54285714 0.55714286 0.57142857 0.58571429 0.6 0.61428571 0.62857143 0.64285714 0.65714286 0.67142857 0.68571429 0.7 0.71428571 0.72857143 0.74285714 0.75714286 0.77142857 0.78571429 0.8 0.81428571 0.82857143 0.84285714 0.85714286 0.87142857 0.88571429 0.9 0.91428571 0.92857143 0.94285714 0.95714286 0.97142857 0.98571429 1 1 1 1 1 1
  arc A6 (6.7857, 18.8137) -> (5.5686, 19.2091) centre (0, 0) ccw
  spline S11 degree 5 poles (6.8081, 15.4838) (6.8117, 15.4922) (6.8188, 15.5089) (6.8287, 15.5342) (6.8406, 15.5685) (6.8536, 15.612) (6.8654, 15.6561) (6.8763, 15.7004) (6.8868, 15.745) (6.897, 15.7896) (6.9069, 15.8344) (6.9163, 15.8793) (6.9252, 15.9245) (6.9335, 15.9698) (6.9411, 16.0154) (6.9481, 16.0611) (6.9546, 16.1071) (6.9607, 16.1532) (6.9664, 16.1994) (6.9717, 16.2457) (6.9767, 16.2921) (6.9813, 16.3387) (6.9855, 16.3854) (6.9892, 16.4321) (6.9926, 16.4791) (6.9956, 16.5261) (6.9982, 16.5732) (7.0004, 16.6205) (7.0024, 16.6678) (7.0039, 16.7152) (7.0052, 16.7627) (7.0061, 16.8103) (7.0066, 16.858) (7.0069, 16.9058) (7.0067, 16.9536) (7.0063, 17.0015) (7.0056, 17.0495) (7.0045, 17.0976) (7.0031, 17.1458) (7.0014, 17.194) (6.9994, 17.2423) (6.9971, 17.2906) (6.9945, 17.339) (6.9916, 17.3875) (6.9884, 17.4361) (6.9849, 17.4847) (6.9811, 17.5333) (6.9771, 17.582) (6.9727, 17.6308) (6.9681, 17.6796) (6.9631, 17.7285) (6.9579, 17.7774) (6.9524, 17.8264) (6.9466, 17.8754) (6.9406, 17.9244) (6.9342, 17.9735) (6.9276, 18.0227) (6.9207, 18.0719) (6.9136, 18.1211) (6.9062, 18.1704) (6.8985, 18.2197) (6.8905, 18.269) (6.8823, 18.3184) (6.8738, 18.3678) (6.8651, 18.4172) (6.8561, 18.4667) (6.8468, 18.5161) (6.8373, 18.5657) (6.8275, 18.6152) (6.8175, 18.6648) (6.8072, 18.7144) (6.7987, 18.7541) (6.7923, 18.7839) (6.7879, 18.8037) (6.7857, 18.8137) knots 0 0 0 0 0 0 0.01428571 0.02857143 0.04285714 0.05714286 0.07142857 0.08571429 0.1 0.11428571 0.12857143 0.14285714 0.15714286 0.17142857 0.18571429 0.2 0.21428571 0.22857143 0.24285714 0.25714286 0.27142857 0.28571429 0.3 0.31428571 0.32857143 0.34285714 0.35714286 0.37142857 0.38571429 0.4 0.41428571 0.42857143 0.44285714 0.45714286 0.47142857 0.48571429 0.5 0.51428571 0.52857143 0.54285714 0.55714286 0.57142857 0.58571429 0.6 0.61428571 0.62857143 0.64285714 0.65714286 0.67142857 0.68571429 0.7 0.71428571 0.72857143 0.74285714 0.75714286 0.77142857 0.78571429 0.8 0.81428571 0.82857143 0.84285714 0.85714286 0.87142857 0.88571429 0.9 0.91428571 0.92857143 0.94285714 0.95714286 0.97142857 0.98571429 1 1 1 1 1 1
  line L11 (6.2595, 14.2336) -> (6.8081, 15.4838)
  line L12 (11.5077, 10.4571) -> (12.5173, 11.3761)
  spline S12 degree 5 poles (12.5173, 11.3761) (12.5241, 11.3822) (12.5373, 11.3946) (12.5567, 11.4137) (12.5815, 11.4402) (12.6111, 11.4747) (12.6397, 11.5101) (12.6678, 11.5462) (12.6955, 11.5826) (12.7229, 11.6193) (12.7502, 11.6562) (12.7771, 11.6934) (12.8036, 11.731) (12.8296, 11.769) (12.855, 11.8076) (12.8801, 11.8465) (12.9047, 11.8859) (12.929, 11.9255) (12.953, 11.9654) (12.9767, 12.0055) (13.0001, 12.0459) (13.0232, 12.0866) (13.0461, 12.1275) (13.0685, 12.1687) (13.0907, 12.2102) (13.1126, 12.252) (13.1341, 12.294) (13.1554, 12.3362) (13.1764, 12.3787) (13.1971, 12.4213) (13.2175, 12.4642) (13.2377, 12.5074) (13.2576, 12.5507) (13.2773, 12.5942) (13.2966, 12.638) (13.3157, 12.6819) (13.3346, 12.7261) (13.3531, 12.7705) (13.3715, 12.815) (13.3895, 12.8597) (13.4074, 12.9047) (13.4249, 12.9498) (13.4422, 12.9951) (13.4593, 13.0405) (13.4761, 13.0862) (13.4927, 13.132) (13.509, 13.178) (13.5251, 13.2242) (13.541, 13.2705) (13.5566, 13.317) (13.572, 13.3636) (13.5871, 13.4104) (13.602, 13.4574) (13.6166, 13.5045) (13.6311, 13.5518) (13.6452, 13.5992) (13.6592, 13.6468) (13.6729, 13.6946) (13.6864, 13.7424) (13.6997, 13.7905) (13.7127, 13.8386) (13.7255, 13.8869) (13.7381, 13.9354) (13.7504, 13.9839) (13.7625, 14.0327) (13.7744, 14.0815) (13.7861, 14.1305) (13.7975, 14.1796) (13.8087, 14.2288) (13.8197, 14.2782) (13.8305, 14.3277) (13.8389, 14.3674) (13.8451, 14.3972) (13.8492, 14.4172) (13.8513, 14.4271) knots 0 0 0 0 0 0 0.01428571 0.02857143 0.04285714 0.05714286 0.07142857 0.08571429 0.1 0.11428571 0.12857143 0.14285714 0.15714286 0.17142857 0.18571429 0.2 0.21428571 0.22857143 0.24285714 0.25714286 0.27142857 0.28571429 0.3 0.31428571 0.32857143 0.34285714 0.35714286 0.37142857 0.38571429 0.4 0.41428571 0.42857143 0.44285714 0.45714286 0.47142857 0.48571429 0.5 0.51428571 0.52857143 0.54285714 0.55714286 0.57142857 0.58571429 0.6 0.61428571 0.62857143 0.64285714 0.65714286 0.67142857 0.68571429 0.7 0.71428571 0.72857143 0.74285714 0.75714286 0.77142857 0.78571429 0.8 0.81428571 0.82857143 0.84285714 0.85714286 0.87142857 0.88571429 0.9 0.91428571 0.92857143 0.94285714 0.95714286 0.97142857 0.98571429 1 1 1 1 1 1
  arc A7 (13.8513, 14.4271) -> (12.9002, 15.2835) centre (0, 0) ccw
  spline S13 degree 5 poles (10.0054, 13.6379) (10.0107, 13.6452) (10.0217, 13.6597) (10.0387, 13.6809) (10.0624, 13.7084) (10.0936, 13.7415) (10.1259, 13.7736) (10.1588, 13.8053) (10.1921, 13.8366) (10.2257, 13.8678) (10.2596, 13.8987) (10.2938, 13.9294) (10.3284, 13.9596) (10.3635, 13.9895) (10.3992, 14.0189) (10.4353, 14.0478) (10.4718, 14.0764) (10.5087, 14.1047) (10.5459, 14.1327) (10.5833, 14.1605) (10.6211, 14.188) (10.6591, 14.2153) (10.6974, 14.2423) (10.736, 14.2689) (10.775, 14.2953) (10.8142, 14.3214) (10.8537, 14.3472) (10.8935, 14.3728) (10.9336, 14.3981) (10.9738, 14.4232) (11.0144, 14.448) (11.0551, 14.4726) (11.0961, 14.4969) (11.1374, 14.521) (11.1789, 14.5448) (11.2206, 14.5684) (11.2625, 14.5918) (11.3047, 14.6149) (11.3471, 14.6378) (11.3897, 14.6604) (11.4325, 14.6828) (11.4756, 14.705) (11.5188, 14.727) (11.5622, 14.7487) (11.6059, 14.7702) (11.6497, 14.7915) (11.6937, 14.8125) (11.738, 14.8333) (11.7824, 14.8539) (11.827, 14.8743) (11.8718, 14.8945) (11.9167, 14.9144) (11.9619, 14.9341) (12.0072, 14.9536) (12.0527, 14.9729) (12.0984, 14.992) (12.1443, 15.0108) (12.1903, 15.0295) (12.2365, 15.0479) (12.2829, 15.0661) (12.3294, 15.0841) (12.3761, 15.1019) (12.423, 15.1194) (12.47, 15.1368) (12.5172, 15.1539) (12.5645, 15.1709) (12.612, 15.1876) (12.6597, 15.2041) (12.7075, 15.2204) (12.7554, 15.2365) (12.8035, 15.2524) (12.8421, 15.2649) (12.8712, 15.2742) (12.8905, 15.2804) (12.9002, 15.2835) knots 0 0 0 0 0 0 0.01428571 0.02857143 0.04285714 0.05714286 0.07142857 0.08571429 0.1 0.11428571 0.12857143 0.14285714 0.15714286 0.17142857 0.18571429 0.2 0.21428571 0.22857143 0.24285714 0.25714286 0.27142857 0.28571429 0.3 0.31428571 0.32857143 0.34285714 0.35714286 0.37142857 0.38571429 0.4 0.41428571 0.42857143 0.44285714 0.45714286 0.47142857 0.48571429 0.5 0.51428571 0.52857143 0.54285714 0.55714286 0.57142857 0.58571429 0.6 0.61428571 0.62857143 0.64285714 0.65714286 0.67142857 0.68571429 0.7 0.71428571 0.72857143 0.74285714 0.75714286 0.77142857 0.78571429 0.8 0.81428571 0.82857143 0.84285714 0.85714286 0.87142857 0.88571429 0.9 0.91428571 0.92857143 0.94285714 0.95714286 0.97142857 0.98571429 1 1 1 1 1 1
  line L13 (9.197, 12.5377) -> (10.0054, 13.6379)
extrude "Extrude4" cut sketch "Sketch7" along normal up to surface (15 mm away) keep common part bodies 4 in component "spur-gear"
extrude "Extrude2'''" cut sketch "Sketch7" along normal up to surface (15 mm away) sketch seen with x (0.943097, 0, 0.332518) y (0.332518, 0, -0.943097) z (0, 1, 0) at (-15.2326, -5, 31.1301) keep common part bodies 5 in component "shaft"
component "spur-gear" placed x (0.943097, 0, 0.332518) y (0.332518, 0, -0.943097) z (0, 1, 0) at (15.9228, 0, 31.5)
component "rack" placed x (1, 0, 0) y (0, 1, 0) z (0, 0, 1) at (0, 0, 0)
component "shaft" placed x (1, 0, 0) y (0, 1, 0) z (0, 0, 1) at (31.1554, 5, 0.3699)
equation "module = 2 mm"
equation "pressureAngle = 20 deg"
equation "teethCount = 7"
equation "lengthOverall = PI * module * teethCount"
equation "rackThickness = 10 mm"
equation "rackWidth = 15 mm"
equation "backlash = 0.15 mm"
equation "d8 = lengthOverall"
equation "d9 = rackThickness"
equation "d10 = 1.25 * module"
equation "d11 = 1 * module"
equation "d12 = 90 deg - pressureAngle"
equation "d13 = PI * module / 2"
equation "d14 = PI * module / 2"
equation "d15 = rackWidth"
equation "d17 = rackWidth"
equation "d20 = 0.38 * module"
equation "d21 = teethCount"
equation "d23 = PI * module"
equation "d32 = 18 mm + 0.75 mm"
equation "d89 = ( 2 * 18 * PI ) * 1 mm"
named bodies: "rack", "rack-top", "spur-gear", "shaft"
